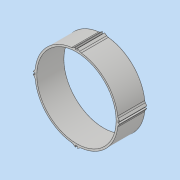
# Autodesk Inventor part: PropShroud
Saved by Autodesk Inventor 2017 (Build 210142000, 142)
## iProperties
Created: 2017-03-05
Part Number: PropShroud
Material: Generic
Document SubType Name: Modeling
Designer: techn
Density: 1 g/cm^3
Appearance: Default
Author: techn
Autodesk Inventor part; units mm, degrees
ref_plane "YZ Plane" through (0, 0, 0) normal (1, 0, 0) x (0, 1, 0)
ref_plane "XZ Plane" through (0, 0, 0) normal (0, 1, 0) x (-1, 0, 0)
ref_plane "XY Plane" through (0, 0, 0) normal (0, 0, 1) x (1, 0, 0)
sketch "Sketch1" plane through (0, 0, 0) normal (0, 0, 1) x (1, 0, 0)
  circle A0 centre (0, 0) radius 14.605
  circle A1 centre (0, 0) radius 13.97
  dimension "d0" = 29.21
  dimension "d1" = 27.94
  constraints: 2 centre point, 2 coincident
  measures "d0" diameter of A0
  measures "d1" diameter of A1
extrude "Extrusion1" add sketch "Sketch1" along normal blind 9.525
sketch "Sketch2" plane through (0, 0, 9.525) normal (0, 0, 1) x (1, 0, 0)
  circle A0 centre (0, 0) radius 13.97 projected
  circle A1 centre (0, 0) radius 14.605 projected
  line L0 (0.381, 14.6) -> (-0.381, 14.6)
  line L1 (0.381, 14.6) -> (0.381, 15.235)
  line L2 (0.381, 15.235) -> (-0.381, 15.235)
  line L3 (-0.381, 15.235) -> (-0.381, 14.6)
  line L4 (-0.381, 15.235) -> (-1.3732, 14.5403)
  line L5 (-0.381, 15.235) -> (0.8302, 15.235) construction
  circle A2 centre (0, 0) radius 14.605 projected
  line L6 (0.381, 15.235) -> (1.3732, 14.5403)
  line L7 (0.381, 15.235) -> (1.5922, 15.235) construction
  dimension "d4" = 0.762
  dimension "d5" = 0.635
  dimension "d8" = 145
  dimension "d9" = 35
  constraints: 16 end point, 4 horizontal, 4 point on circle, 2 equal length, 1 perpendicular, 1 vertical
  measures "d4" distance of L0.start L0.end
  measures "d5" distance of L0.start L1.end
  measures "d8" angle of L4 L5
  measures "d9" angle of L6 L7
extrude "Extrusion2" add sketch "Sketch2" against normal blind 9.525 contours A1 L1 L6 | L4 L3 A1
fillet "Fillet1" radius 1.27 2 edges at (1.3732, 14.5403, 4.7625) (-1.3732, 14.5403, 4.7625)
pattern_circular "Circular Pattern1" count 4 over 360 about axis through (0, 0, 0) along (0, 0, 1) of "Extrusion2", "Fillet1"
body "Solid1"
